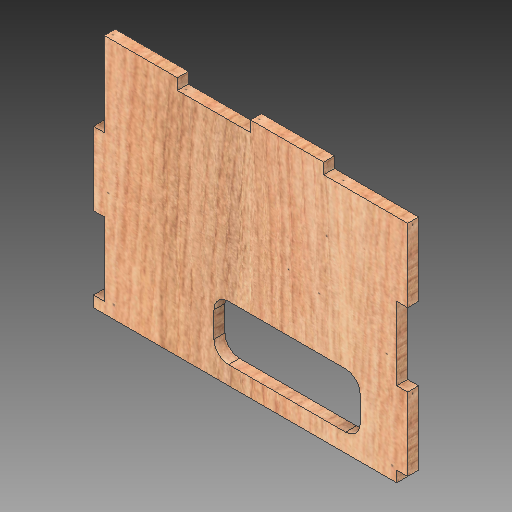
# Autodesk Inventor part: ControlBoxSide
Saved by Autodesk Inventor 2018.2 (Build 222227000, 227)
## iProperties
Created: 2018-03-30
Part Number: ControlBoxSide
Material: Wood (Birch)
Document SubType Name: Modeling
Designer: Muchen He
Density: 0.55 g/cm^3
Appearance: Birch - Natural Polished
Mass: 7.85851 g
Surface Area: 108.009 cm^2
Volume: 14.2882 cm^3
Author: Muchen He
Autodesk Inventor part; units mm, degrees
ref_plane "YZ Plane" through (0, 0, 0) normal (1, 0, 0) x (0, 1, 0)
ref_plane "XZ Plane" through (0, 0, 0) normal (0, 1, 0) x (-1, 0, 0)
ref_plane "XY Plane" through (0, 0, 0) normal (0, 0, 1) x (1, 0, 0)
sketch "Sketch1" plane through (0, 0, 0) normal (0, 0, 1) x (1, 0, 0)
  line L0 (0, 0) -> (83, 0)
  line L1 (0, 0) -> (0, 3)
  line L2 (0, 3) -> (3, 3)
  line L3 (3, 3) -> (3, 23)
  line L4 (3, 23) -> (0, 23)
  line L5 (0, 23) -> (0, 43)
  line L6 (0, 43) -> (3, 43)
  line L7 (3, 43) -> (3, 63)
  line L8 (3, 63) -> (3, 66)
  line L9 (3, 66) -> (23, 66)
  line L10 (23, 66) -> (23, 63)
  line L11 (23, 63) -> (43, 63)
  line L12 (43, 63) -> (43, 66)
  line L13 (43, 66) -> (63, 66)
  line L14 (63, 66) -> (63, 63)
  line L15 (63, 63) -> (83, 63)
  line L16 (83, 63) -> (86, 63)
  line L17 (86, 63) -> (86, 43)
  line L18 (86, 43) -> (83, 43)
  line L19 (83, 43) -> (83, 23)
  line L20 (83, 23) -> (86, 23)
  line L21 (86, 23) -> (86, 3)
  line L22 (83, 3) -> (83, 0)
  line L23 (83, 3) -> (86, 3)
  dimension "d0" = 83
  dimension "d1" = 3
  dimension "d2" = 3
  dimension "d3" = 20
  dimension "d4" = 20
  dimension "d5" = 20
  dimension "d6" = 3
  dimension "d7" = 20
  dimension "d8" = 20
  dimension "d9" = 20
  dimension "d10" = 20
  dimension "d11" = 3
  dimension "d12" = 20
  dimension "d13" = 3
  dimension "d14" = 20
  dimension "d16" = 20
  constraints: 48 end point, 13 perpendicular, 7 point on line, 5 vertical, 3 horizontal, 1 horizontal alignment, 1 vertical alignment
  measures "d0" distance of L0.start L0.end
  measures "d1" distance of L0.start L1.end
  measures "d2" distance of L1.end L2.end
  measures "d3" distance of L2.end L3.end
  measures "d4" distance of L4.end L5.end
  measures "d5" distance of L6.end L7.end
  measures "d6" distance of L7.end L8.end
  measures "d7" distance of L8.end L9.end
  measures "d8" distance of L10.end L11.end
  measures "d9" distance of L12.end L13.end
  measures "d10" distance of L14.end L15.end
  measures "d11" distance of L15.end L16.end
  measures "d12" distance of L16.end L17.end
  measures "d13" distance of L17.end L18.end
  measures "d14" distance of L18.end L19.end
  measures "d16" distance of L20.end L21.end
extrude "Extrusion1" add sketch "Sketch1" along normal blind 3
sketch "Sketch2" plane through (0, 0, 3) normal (0, 0, 1) x (1, 0, 0)
  line L0 (33, 20) -> (73, 20)
  line L1 (73, 20) -> (73, 5)
  line L2 (73, 5) -> (33, 5)
  line L3 (33, 5) -> (33, 20)
  line L4 (0, 0) -> (83, 0) projected
  line L5 (83, 23) -> (83, 43) projected
  dimension "d19" = 5
  dimension "d20" = 10
  dimension "d21" = 15
  dimension "d22" = 40
  constraints: 8 end point, 2 parallel, 1 horizontal, 1 perpendicular
  measures "d19" distance between parallel lines of L4 L2
  measures "d20" distance between parallel lines of L5 L1
  measures "d21" distance of L2.end L0.start
  measures "d22" distance of L1.end L2.end
extrude "Extrusion2" cut sketch "Sketch2" against normal through all
fillet "Fillet1" radius 4 4 edges at (73, 5, 1.5) (73, 20, 1.5) (33, 20, 1.5) (33, 5, 1.5)
body "Solid1"
